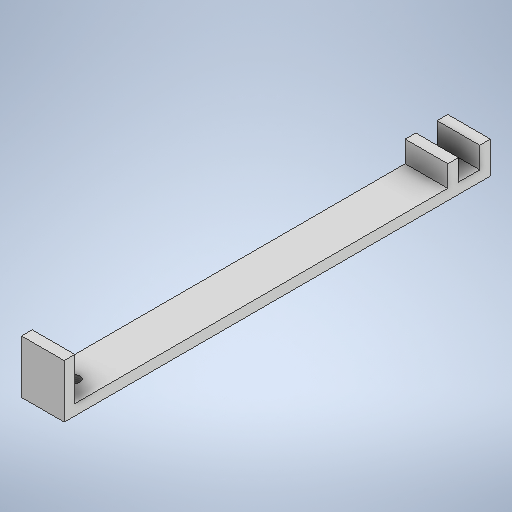
# Autodesk Inventor part: Conexión - C15
Saved by Autodesk Inventor 2025.3 (Build 293356000, 356)
## iProperties
Created: 2025-11-24
Part Number: Conexión - C15
Material: Genérico
Document SubType Name: Modeling
Designer: Gianluca Nuñez
Density: 1 g/cm^3
Appearance: Valor por defecto
Author: Gianluca Nuñez
## iProperties of the stored document Conexión - C15_3DPrint.ipt
Created: 2025-11-24
Part Number: Conexión - C15_3DPrint
Material: Genérico
Document SubType Name: Modeling
Designer: Gianluca Nuñez
Density: 1 g/cm^3
Appearance: Valor por defecto
Author: Gianluca Nuñez
Autodesk Inventor part; units mm, degrees
ref_plane "YZ Plane" through (0, 0, 0) normal (1, 0, 0) x (0, 1, 0)
ref_plane "XZ Plane" through (0, 0, 0) normal (0, 1, 0) x (-1, 0, 0)
ref_plane "XY Plane" through (0, 0, 0) normal (0, 0, 1) x (1, 0, 0)
sketch "Boceto1" plane through (0, 0, 0) normal (0, 0, 1) x (1, 0, 0)
  line L0 (0, 0) -> (-20, 0)
  line L1 (-20, 0) -> (-20, -5)
  line L2 (-20, -5) -> (0, -5)
  line L3 (0, -5) -> (0, 0)
  dimension "d0" = 20
  dimension "d1" = 5
  constraints: 8 end point, 2 parallel, 1 horizontal, 1 perpendicular
  measures "d0" distance of L2.end L1.end
  measures "d1" distance of L0.end L1.end
extrude "Extrusión1" add sketch "Boceto1" along normal blind 200
sketch "Boceto2" plane through (-20, 0, 0) normal (0, 1, 0) x (1, 0, 0)
  circle A0 centre (10, -185) radius 2.5
  circle A1 centre (10, -10) radius 2.5
  line L0 (0, 0) -> (0, -200) projected
  line L1 (0, -15) -> (20, -15) construction
  line L2 (20, 0) -> (0, 0) construction
  dimension "d4" = 5
  dimension "d5" = 5
  dimension "d6" = 10
  dimension "d7" = 10
  dimension "d8" = 15
  dimension "d9" = 10
  dimension "d10" = 170
  constraints: 2 centre point, 2 end point, 1 horizontal, 1 point on line
  measures "d4" diameter of A0
  measures "d5" diameter of A1
  measures "d6" distance from line of L0 A1.centre
  measures "d7" distance from line of L0 A0.centre
  measures "d8" distance between parallel lines of L2 L1
  measures "d9" distance from line of L2 A1.centre
  measures "d10" distance from line of A0.centre L1
extrude "Extrusión2" cut sketch "Boceto2" against normal blind 200
sketch "Boceto3" plane through (-20, 0, 0) normal (0, 1, 0) x (1, 0, 0)
  line L0 (20, -200) -> (0, -200) projected
  line L1 (20, 0) -> (20, -200) projected
  line L2 (0, -200) -> (20, -200)
  line L3 (20, -200) -> (20, -195)
  line L4 (20, -195) -> (0, -195)
  line L5 (0, -195) -> (0, -200)
  dimension "d13" = 5
  constraints: 8 end point, 2 parallel, 1 horizontal, 1 perpendicular, 1 point on line
  measures "d13" distance of L3.end L2.end
extrude "Extrusión3" add sketch "Boceto3" along normal blind 20
sketch "Boceto4" plane through (-20, 0, 0) normal (0, 1, 0) x (1, 0, 0)
  line L0 (20, 0) -> (20, -200) projected
  line L1 (0, 0) -> (20, 0)
  line L2 (20, 0) -> (20, -5)
  line L3 (20, -5) -> (0, -5)
  line L4 (0, -5) -> (0, 0)
  line L5 (0, 0) -> (0, -200) projected
  line L6 (0, -15) -> (20, -15)
  line L7 (20, -15) -> (20, -20)
  line L8 (20, -20) -> (0, -20)
  line L9 (0, -20) -> (0, -15)
  dimension "d16" = 5
  dimension "d17" = 5
  dimension "d18" = 10
  constraints: 16 end point, 4 parallel, 3 point on line, 2 horizontal, 2 perpendicular
  measures "d16" distance of L1.end L2.end
  measures "d17" distance of L6.end L7.end
  measures "d18" distance between parallel lines of L3 L6
extrude "Extrusión4" add sketch "Boceto4" along normal blind 10 contours L0 L3 L4 L1 | L0 L8 L5 L6
thread "Rosca1" size "M5x0.8" class "6H" standard "ANSI Metric M Profile" full length
thread "Rosca2" size "M5x0.8" class "6H" standard "ANSI Metric M Profile" full length
